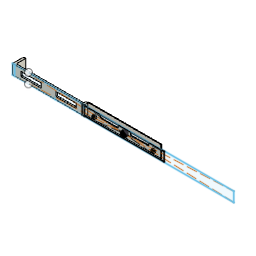
A4フレーム v8 (Autodesk Fusion 360 design; units mm, degrees)
Autodesk Fusion 360 part; units mm, degrees
note: some values were not read from the file. Set by a fixed rule: which face or edge a step refers to.
sketch "スケッチ1" plane through (0, 0, 0) normal (0, 1, 0) x (1, 0, 0)
  line L0 (148.5, 77.3125) -> (-148.5, 77.3125)
  line L1 (-148.5, 77.3125) -> (-148.5, -132.6875)
  line L2 (148.5, -132.6875) -> (148.5, 77.3125)
  circle A0 centre (-40, -120.6875) radius 3
  circle A1 centre (40, -120.6875) radius 3
  line L3 (0, -132.6875) -> (-0.0009, -17.6875)
  line L4 (-0.0009, -17.6875) -> (139.9991, -17.6875)
  line L5 (-0.0009, -17.6875) -> (-140.0009, -17.6875)
  line L6 (-0.0009, -17.6875) -> (0, 77.3125)
  line L7 (139.9991, -17.6875) -> (148.5, -17.6875)
  line L8 (-140.0009, -17.6875) -> (-148.5, -17.6875)
  line L9 (-127.0009, -132.6875) -> (-127.0009, -115.6875)
  line L10 (-127.0009, -120.6875) -> (-122.0009, -120.6875)
  line L11 (-127.0009, -120.6875) -> (-132.0009, -120.6875)
  line L12 (127.0009, -132.6855) -> (127.0007, -115.6855)
  line L13 (127.0007, -120.6855) -> (122.0007, -120.6855)
  line L14 (127.0007, -120.6855) -> (132.0007, -120.6854)
  line L15 (108.3724, 43.2725) -> (-108.3743, 43.2725)
  line L16 (-108.3743, 43.2725) -> (-108.3743, -78.6475)
  line L17 (-108.3743, -78.6475) -> (108.3724, -78.6475)
  line L18 (108.3724, -78.6475) -> (108.3724, 43.2725)
  line L19 (126.9991, 63.2538) -> (-127.0009, 63.2538)
  line L20 (-127.0009, 63.2538) -> (-127.0009, -98.6289)
  line L21 (-127.0009, -98.6289) -> (126.9991, -98.6289)
  line L22 (126.9991, -98.6289) -> (126.9991, 63.2538)
  point P0 (-0.0009, -17.6875)
  point P1 (-0.0009, -17.6875)
  point P2 (-0.0009, -17.6875)
  point P3 (-0.0009, -17.6875)
  point P4 (-0.0009, -17.6875)
  dimension "d1" = 297
  dimension "d2" = 210
  dimension "d5" = 6
  dimension "d6" = 6
  dimension "d22" = 115
  dimension "d52" = 17
  dimension "d54" = 5
  dimension "d55" = 5
  dimension "d56" = 216.7467
  dimension "d57" = 121.92
  dimension "d58" = 254
  dimension "d59" = 161.8827
  constraint horizontal L0
  constraint perpendicular L0 L1
  constraint parallel L1 L2
  constraint coincident P4 P3
  constraint midpoint L0 L6.end
  constraint coincident L2 L7.end
  constraint perpendicular L2 L7
  constraint coincident L1 L8.end
  constraint perpendicular L1 L8
  constraint coincident L9 L10.start
  constraint perpendicular L9 L10
  constraint perpendicular L9 L11
  constraint symmetric L3 L9.start L12.start
  constraint symmetric L3 L9.end L12.end
  constraint symmetric L3 L10.start L13.start
  constraint symmetric L3 L10.end L13.end
  constraint symmetric L3 L11.end L14.end
  constraint horizontal L15
  constraint perpendicular L15 L16
  constraint parallel L15 L17
  constraint parallel L16 L18
  constraint horizontal L19
  constraint perpendicular L19 L20
  constraint parallel L19 L21
  constraint parallel L20 L22
  measures "d1" distance of L1.end L2.start
  measures "d2" distance of L0.end L1.end
  measures "d5" diameter of A0
  measures "d6" diameter of A1
  measures "d22" vertical distance of L3.start P4
  measures "d52" distance of L9.start L9.end
  measures "d54" distance of L10.start L10.end
  measures "d55" distance of L10.start L11.end
  measures "d56" distance of L16.end L17.end
  measures "d57" distance of L15.end L16.end
  measures "d58" distance of L20.end L21.end
  measures "d59" distance of L19.end L20.end
sketch "スケッチ2" plane through (0, 0, 0) normal (0, 1, 0) x (1, 0, 0)
  line L0 (-148.5, 77.3125) -> (-148.5, -132.6875)
  line L1 (148.5, 77.3125) -> (-148.5, 77.3125)
  line L2 (148.5, -132.6875) -> (148.5, 77.3125)
  line L3 (-88.4729, -129.9233) -> (-88.4729, -114.7866)
  line L4 (-95.2664, -123.6333) -> (-107.9664, -123.6333)
  line L5 (-88.4729, -114.7866) -> (-116.5039, -114.7866)
  line L6 (-116.5039, -114.7866) -> (-116.5039, -129.9233)
  line L7 (107.9501, -123.6333) -> (95.2501, -123.6333)
  line L8 (-116.5039, -129.9233) -> (-88.4729, -129.9233)
  line L9 (8.7983, -129.9233) -> (8.7983, -115.0112)
  line L10 (-8.7981, -129.9233) -> (8.7983, -129.9233)
  line L11 (95.2501, -120.4583) -> (107.9501, -120.4583)
  spline S0 degree 3 poles (107.9501, -120.4583) (108.8269, -120.4583) (109.5376, -121.1691) (109.5376, -122.0458) (109.5376, -122.9226) (108.8269, -123.6333) (107.9501, -123.6333) knots 1 1 1 1 2 2 2 3 3 3 3
  line L12 (88.4567, -129.9233) -> (116.4876, -129.9233)
  line L13 (116.4876, -114.7866) -> (88.4567, -114.7866)
  line L14 (116.4876, -129.9233) -> (116.4876, -114.7866)
  spline S1 degree 3 poles (95.2501, -123.6333) (94.3733, -123.6333) (93.6626, -122.9226) (93.6626, -122.0458) (93.6626, -121.1691) (94.3733, -120.4583) (95.2501, -120.4583) knots 4 4 4 4 5 5 5 6 6 6 6
  spline S2 degree 3 poles (-107.9664, -123.6333) (-108.8432, -123.6333) (-109.5539, -122.9226) (-109.5539, -122.0458) (-109.5539, -121.1691) (-108.8432, -120.4583) (-107.9664, -120.4583) knots 4 4 4 4 5 5 5 6 6 6 6
  spline S3 degree 3 poles (-95.2664, -120.4583) (-94.3897, -120.4583) (-93.6789, -121.1691) (-93.6789, -122.0458) (-93.6789, -122.9226) (-94.3897, -123.6333) (-95.2664, -123.6333) knots 1 1 1 1 2 2 2 3 3 3 3
  line L15 (-107.9664, -120.4583) -> (-95.2664, -120.4583)
  line L16 (8.7983, -115.0112) -> (-8.7981, -115.0112)
  line L17 (88.4567, -114.7866) -> (88.4567, -129.9233)
  line L18 (-8.7981, -115.0112) -> (-8.7981, -129.9233)
  circle A0 centre (0.0001, -122.0458) radius 3.175
  dimension "d25" = 297
  dimension "d26" = 210
  dimension "d51" = 6.35
  constraint horizontal L1
  constraint perpendicular L0 L1
  constraint parallel L0 L2
  measures "d25" distance of L2.start L0.end
  measures "d26" distance of L0.end L0.start
  measures "d51" diameter of A0
sketch "スケッチ4" plane through (0, 0, 0) normal (0, 1, 0) x (1, 0, 0)
  line L0 (40, -0.0125) -> (-40, -0.0125)
  circle A0 centre (-40, -0.0125) radius 3
  circle A1 centre (40, -0.0125) radius 3
  line L1 (50, 5) -> (-50, 5)
  line L2 (-50, 5) -> (-50, -5)
  line L3 (-50, -5) -> (50, -5)
  line L4 (50, -5) -> (50, 5)
  line L5 (50, 5) -> (-50, -5) construction
  line L6 (-50, 5) -> (50, -5) construction
  dimension "d27" = 6
  dimension "d28" = 6
  dimension "d29" = 100
  dimension "d30" = 10
  constraint horizontal L0
  constraint coincident L0.end A0.centre
  constraint coincident L0.start A1.centre
  constraint horizontal L1
  constraint perpendicular L1 L2
  constraint parallel L1 L3
  constraint parallel L2 L4
  constraint coincident L5 origin
  constraint coincident L6 origin
  measures "d27" diameter of A0
  measures "d28" diameter of A1
  measures "d29" distance of L2.end L3.end
  measures "d30" distance of L1.end L2.end
extrude "押し出し1" add sketch "スケッチ4" along normal blind 0.9 contours A0 | A1 | L1 L2 L3 L4 makes body 1
extrude "押し出し2" add sketch "スケッチ4" against normal blind 8 contours A0 | A1 bodies 1
chamfer "面取り1" distance 1 angle 45 2 edges at (-42.797, -8, -1.0723) (37.203, -8, -1.0723) on bodies 1
chamfer "面取り2" distance 0.5 angle 45 1 faces at (-47.6667, 0, 0.0042) on bodies 1
sketch "スケッチ5" plane through (0, 0.9, 0) normal (0, 1, 0) x (-1, 0, 0)
  line L0 (-50, 5) -> (-50, -5)
  line L1 (-50, -5) -> (50, -5)
  line L2 (50, -5) -> (50, 5)
  line L3 (50, 5) -> (-50, 5)
  line L4 (-33, 2) -> (33, 2)
  line L5 (33, 2) -> (33, -2)
  line L6 (33, -2) -> (-33, -2)
  line L7 (-33, -2) -> (-33, 2)
  line L8 (-33, 2) -> (33, -2) construction
  line L9 (33, 2) -> (-33, -2) construction
  line L10 (-8.3796, 2) -> (8.3796, 2)
  line L11 (8.3796, 2) -> (8.3796, -2)
  line L12 (8.3796, -2) -> (-8.3796, -2)
  line L13 (-8.3796, -2) -> (-8.3796, 2)
  line L14 (-8.3796, 2) -> (8.3796, -2) construction
  line L15 (8.3796, 2) -> (-8.3796, -2) construction
  constraint horizontal L4
  constraint perpendicular L4 L5
  constraint parallel L4 L6
  constraint parallel L5 L7
  constraint coincident L8 origin
  constraint coincident L9 origin
  constraint horizontal L10
  constraint perpendicular L10 L11
  constraint parallel L10 L12
  constraint parallel L11 L13
  constraint coincident L14 origin
  constraint coincident L15 origin
  constraint coincident L4 L10.start
extrude "押し出し3" cut sketch "スケッチ5" against normal blind 8 contours L4 L6 L7 L13 | L4 L5 L6 L11 bodies 1
delete_face "面を削除1" 1 faces at (-36.6708, -0.1667, 0.1787) on bodies 1
delete_face "面を削除2" 1 faces at (43.3168, -0.1667, -0.3194) on bodies 1
sketch "スケッチ6" plane through (0, -8, 0) normal (0, -1, 0) x (1, 0, 0)
  circle A0 centre (-40, 0.0125) radius 2
  circle A1 centre (-40, 0.0125) radius 1
  circle A2 centre (40, 0) radius 1
  dimension "d39" = 2
  dimension "d40" = 2
  constraint concentric A0 A1
  measures "d39" diameter of A1
  measures "d40" diameter of A2
extrude "押し出し4" cut sketch "スケッチ6" against normal blind 15 contours A1 | A2 bodies 1
move_face "面をオフセット1" offset -0.4 1 faces at (-37.0037, -4.6667, 0.162) on bodies 1
move_face "面をオフセット2" offset -0.4 1 faces at (42.9851, -4.6667, 0.3112) on bodies 1
move_face "面を移動1" by (0, 0.36, 0) 1 faces at (47, 0.9, 0) on bodies 1
move_face "面を移動2" to x (1, 0, 0) y (0, 1, 0) z (0, 0, 1) at (0, 2, 0) 4 faces at (-38.606, -8, -0.067) (-40.8281, -7.3333, -2.0975) (39.4167, -8, 1.277) (40.5044, -7.3333, -2.1973) on bodies 1
copy_body "ボディのコピーと貼り付け1" bodies 1 makes body 2
move_face "面を移動3" by (0, -0.4, 0) 1 faces at (47, 1.26, 0) on bodies 2
delete_face "面を削除3" 1 faces at (40.5044, -5.3333, -2.1973) on bodies 2
delete_face "面を削除4" 1 faces at (-40.8281, -5.3333, -2.0975) on bodies 2
move_face "面を移動4" by (0, 4, 0) 2 faces at (-37.943, -6, 0.1417) (40.5837, -6, 1.985) on bodies 2
move_face "面を移動5" by (0, 0.5, 0) 2 faces at (-37.943, -2, 0.1417) (40.5837, -2, 1.985) on bodies 2
chamfer "面取り3" distance 0.5 angle 45 2 edges at (-42.4241, -1.5, 0.9527) (37.5759, -1.5, 0.9527) on bodies 2
move_face "面を移動6" to x (1, 0, 0) y (0, 1, 0) z (0, 0, 1) at (0, -0.5, 0) 4 faces at (-41.1939, -1.5, 1.2626) (-37.5788, -1.1667, 0.2548) (42.4212, -1.1667, 0.2548) (40.4857, -1.5, 1.6674) on bodies 2
sketch "スケッチ7" plane through (0, 0.86, 0) normal (0, 1, 0) x (-1, 0, 0)
  circle A0 centre (40, 0.0125) radius 1
  circle A1 centre (-40, 0) radius 1
  line L0 (8.3796, -2) -> (8.3796, 2)
  line L1 (8.3796, 2) -> (33, 2)
  line L2 (33, 2) -> (33, -2)
  line L3 (33, -2) -> (8.3796, -2)
  line L4 (-8.3796, 2) -> (-8.3796, -2)
  line L5 (-8.3796, -2) -> (-33, -2)
  line L6 (-33, -2) -> (-33, 2)
  line L7 (-33, 2) -> (-8.3796, 2)
  line L8 (-50, 5) -> (-50, -5)
  line L9 (-50, -5) -> (50, -5)
  line L10 (50, -5) -> (50, 5)
  line L11 (50, 5) -> (-50, 5)
  line L12 (0, 0) -> (0, 5)
  line L13 (0, 12) -> (50, 12)
  line L14 (50, 12) -> (50, 5)
  line L15 (0, 12) -> (-50, 12)
  line L16 (-50, 12) -> (-50, 5)
  line L17 (-50, 5) -> (50, 5)
  dimension "d62" = 12
  constraint coincident L12.start origin
  constraint perpendicular L11 L12
  constraint perpendicular L12 L13
  constraint coincident L10.end L11.start
  constraint perpendicular L11 L14
  constraint perpendicular L12 L15
  constraint coincident L8.start L11.end
  constraint perpendicular L11 L16
  constraint coincident L11 L12.end
  measures "d62" distance of L12.start L13.start
delete_face "面を削除5" 1 faces at (-16.5, 0.3333, 4.8333) on bodies 2
delete_face "面を削除6" 1 faces at (49.8333, 0.3333, -1.5) on bodies 2
delete_face "面を削除7" 1 faces at (-49.8333, 0.3333, -1.5) on bodies 2
extrude "押し出し5" add sketch "スケッチ7" against normal blind 0.86 contours L11 L13 L14 L15 L16 L17 bodies 2
move_face "面を移動7" by (0, 0, 4) 4 faces at (-16.5864, 0.5733, 2) (24.7932, 0.5733, 2) (-24.7932, 0.5733, -2) (16.5864, 0.5733, -2) on bodies 2
chamfer "面取り4" distance 0.5 angle 45 2 edges at (-50, 0, 3.75) (50, 0, 3.75) on bodies 2
sketch "スケッチ8" plane through (0, 0, 0) normal (0, 1, 0) x (1, 0, 0)
  line L0 (148.5, 6.6742) -> (-151.5, 6.6742)
  line L1 (-148.5, 6.6742) -> (-148.5, -6.6742)
  line L2 (-148.5, -6.6742) -> (148.5, -6.6742)
  line L3 (148.5, -6.6742) -> (148.5, 6.6742)
  line L4 (148.5, 6.6742) -> (-148.5, -6.6742) construction
  line L5 (-148.5, 6.6742) -> (148.5, -6.6742) construction
  line L6 (54, 6) -> (-54, 6)
  line L7 (-54, 6.6742) -> (-54, -6.6742)
  line L8 (-54, -6) -> (54, -6)
  line L9 (54, -6) -> (54, 6)
  line L10 (54, 6) -> (-54, -6) construction
  line L11 (-54, 6) -> (54, -6) construction
  line L12 (-130, 6.8044) -> (-130, 5.8427)
  line L13 (-130, -5.8427) -> (-130, -6.8044)
  line L14 (-93.75, 4.2135) -> (-93.75, 6.6742)
  line L15 (-148.5, -6.6742) -> (-151.5, -6.6742)
  line L16 (-151.5, -6.6742) -> (-151.5, 6.6742)
  line L17 (-148.5, 6.6742) -> (-148.5, -6.6742)
  line L18 (-54, -3.4216) -> (-57, -3.4216)
  line L19 (-57, -6.6742) -> (-57, 6.6742)
  dimension "d66" = 297
  dimension "d67" = 108
  dimension "d68" = 12
  dimension "d77" = 3
  dimension "d79" = 3
  constraint horizontal L0
  constraint perpendicular L0 L1
  constraint parallel L0 L2
  constraint parallel L1 L3
  constraint coincident L4 origin
  constraint coincident L5 origin
  constraint horizontal L6
  constraint perpendicular L6 L7
  constraint parallel L6 L8
  constraint parallel L7 L9
  constraint coincident L10 origin
  constraint coincident L11 origin
  constraint coincident L5 L12.end
  constraint coincident L4 L13.start
  constraint collinear L12 L13
  constraint coincident L0 L14.end
  constraint perpendicular L0 L14
  constraint coincident L5 L14.start
  constraint coincident L2 L7.end
  constraint coincident L8.start L7
  constraint coincident L0 L7.start
  constraint coincident L6.end L7
  constraint horizontal L15
  constraint vertical L16
  constraint vertical L17
  constraint coincident L1.start L0
  constraint coincident L7 L18.start
  constraint perpendicular L7 L18
  constraint coincident L0 L19.end
  constraint perpendicular L0 L19
  constraint coincident L18.end L19
  constraint coincident L2 L19.start
  measures "d66" distance of L1.end L2.end
  measures "d67" distance of L8.start L8.end
  measures "d68" distance of L6.end L8.start
  measures "d77" distance of L1.end L15.end
  measures "d79" distance of L18.start L18.end
extrude "押し出し6" add sketch "スケッチ8" along normal blind 1 separate body contours L0 L7 L18 L19 | L0 L1 L2 L17 L19 | L2 L7 L18 L19 makes body 3
extrude "押し出し7" add sketch "スケッチ8" against normal blind 10 contours L0 L1 L2 L17 L19 | L2 L7 L18 L19 | L0 L1 L15 L16 L17 bodies 3
sketch "スケッチ9" plane through (0, 0, 0) normal (0, -1, 0) x (1, 0, 0)
  line L0 (-57, -6.6742) -> (-54, -6.6742)
  line L1 (-55.5, 5.3258) -> (-55.5, -6.6742)
  line L2 (-24.75, -3.6742) -> (-86.25, -3.6742)
  line L3 (-86.25, -3.6742) -> (-86.25, 2.3258)
  line L4 (-86.25, 2.3258) -> (-24.75, 2.3258)
  line L5 (-24.75, 2.3258) -> (-24.75, -3.6742)
  line L6 (-24.75, -3.6742) -> (-86.25, 2.3258) construction
  line L7 (-86.25, -3.6742) -> (-24.75, 2.3258) construction
  line L8 (-50.75, -3.6742) -> (-60.25, -3.6742)
  line L9 (-60.25, -3.6742) -> (-60.25, 2.3258)
  line L10 (-60.25, 2.3258) -> (-50.75, 2.3258)
  line L11 (-50.75, 2.3258) -> (-50.75, -3.6742)
  line L12 (-50.75, -3.6742) -> (-60.25, 2.3258) construction
  line L13 (-60.25, -3.6742) -> (-50.75, 2.3258) construction
  line L14 (-57, 3.4216) -> (-57, -6.6742)
  line L15 (-54, -6.6742) -> (-54, 3.4216)
  line L16 (-54, 3.4216) -> (-57, 3.4216)
  point P0 (-55.5, -0.6742)
  point P1 (-55.5, -0.6742)
  constraint midpoint L0 L1.end
  constraint horizontal L2
  constraint perpendicular L2 L3
  constraint parallel L2 L4
  constraint parallel L3 L5
  constraint coincident L6 P1
  constraint coincident L7 P1
  constraint midpoint L1 P1
  constraint horizontal L8
  constraint perpendicular L8 L9
  constraint parallel L8 L10
  constraint parallel L9 L11
  constraint coincident L12 P1
  constraint coincident L13 P1
  constraint coincident L2 L8.start
  constraint coincident P1 P0
extrude "押し出し8" cut sketch "スケッチ9" against normal blind 7 contours L2 L3 L4 L9 | L2 L4 L5 L11 bodies 3
move_face "面を移動8" [no effect]
move_face "面を移動9" [no effect]
delete_body "RemoveBody1" bodies 3
extrude "押し出し9" add sketch "スケッチ8" along normal blind 15 separate body contours L0 L7 L18 L19 | L2 L7 L18 L19 | L0 L1 L15 L16 L17 makes body 4 at (-148.5, 10, -2.2247) makes body 5 at (-54, 10, -2.2247)
extrude "押し出し10" add sketch "スケッチ8" along normal blind 2 contours L0 L1 L2 L17 L19 bodies 4 5
move_face "面を移動10" by (0, -5, 0) 1 faces at (-55, 15, -2.2247) on bodies 4
sketch "スケッチ10" plane through (0, 2, 0) normal (0, 1, 0) x (-1, 0, 0)
  line L0 (57, 6.6742) -> (57, -6.6742)
  line L1 (57, -6.6742) -> (148.5, -6.6742)
  line L2 (148.5, -6.6742) -> (148.5, 6.6742)
  line L3 (148.5, 6.6742) -> (57, 6.6742)
  line L4 (102.75, -6.6742) -> (102.75, 6.6742)
  line L5 (65.25, 3) -> (140.25, 3)
  line L6 (140.25, 3) -> (140.25, -3)
  line L7 (140.25, -3) -> (65.25, -3)
  line L8 (65.25, -3) -> (65.25, 3)
  line L9 (65.25, 3) -> (140.25, -3) construction
  line L10 (140.25, 3) -> (65.25, -3) construction
  line L11 (92.75, 4) -> (112.75, 4)
  line L12 (112.75, 4) -> (112.75, -4)
  line L13 (112.75, -4) -> (92.75, -4)
  line L14 (92.75, -4) -> (92.75, 4)
  line L15 (92.75, 4) -> (112.75, -4) construction
  line L16 (112.75, 4) -> (92.75, -4) construction
  point P0 (102.75, 0)
  point P1 (102.75, 0)
  dimension "d84" = 75
  dimension "d85" = 6
  dimension "d86" = 20
  constraint midpoint L1 L4.start
  constraint midpoint L3 L4.end
  constraint horizontal L5
  constraint perpendicular L5 L6
  constraint parallel L5 L7
  constraint parallel L6 L8
  constraint coincident L9 P1
  constraint coincident L10 P1
  constraint midpoint L4 P1
  constraint horizontal L11
  constraint perpendicular L11 L12
  constraint parallel L11 L13
  constraint parallel L12 L14
  constraint coincident L15 P1
  constraint coincident L16 P1
  constraint coincident P1 P0
  measures "d84" distance of L6.end L7.end
  measures "d85" distance of L5.end L6.end
  measures "d86" distance of L12.end L13.end
extrude "押し出し11" cut sketch "スケッチ10" against normal blind 26 contours L5 L7 L8 L14 | L5 L6 L7 L12 bodies 4
chamfer "面取り5" distance 1 angle 45 1 edges at (-57, 2, 0) on bodies 4
chamfer "面取り6" distance 1 angle 45 1 edges at (-148.5, 2, 0) on bodies 4
move_face "面を移動11" by (0, -5, 0) 1 faces at (-55, 10, -2.2247) on bodies 4
chamfer "面取り7" distance 1 angle 45 1 edges at (-151.5, 15, 0) on bodies 4
hidden bodies 1
named bodies: "二ツ穴タップ", "二ツ穴タップ_scan", "パンチサポート", "二ツ穴サポート"
